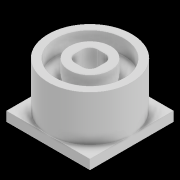
# Autodesk Inventor part: Boton Base
Saved by Autodesk Inventor 2020 (Build 240168000, 168)
## iProperties
Created: 2022-02-20
Part Number: Boton Base
Material: Genérico
Document SubType Name: Modeling
Designer: Alférez
Density: 1 g/cm^3
Appearance: Valor por defecto
Author: Alférez
Autodesk Inventor part; units mm, degrees
ref_plane "YZ Plane" through (0, 0, 0) normal (1, 0, 0) x (0, 1, 0)
ref_plane "XZ Plane" through (0, 0, 0) normal (0, 1, 0) x (-1, 0, 0)
ref_plane "XY Plane" through (0, 0, 0) normal (0, 0, 1) x (1, 0, 0)
sketch "Boceto1" plane through (0, 0, 0) normal (0, 1, 0) x (-1, 0, 0)
  line L0 (0, 0) -> (11, 0)
  line L1 (11, 0) -> (11, -11)
  line L2 (11, -11) -> (0, -11)
  line L3 (0, -11) -> (0, 0)
  dimension "d0" = 11
  dimension "d1" = 11
  constraints: 8 end point, 2 parallel, 1 horizontal, 1 perpendicular
  measures "d0" distance of L1.end L2.end
  measures "d1" distance of L0.end L1.end
extrude "Extrusión1" add sketch "Boceto1" along normal blind 1.25
sketch "Boceto2" plane through (0, 1.25, 0) normal (0, 1, 0) x (1, 0, 0)
  line L0 (-11, 0) -> (0, 0) projected
  line L1 (-11, 11) -> (-11, 0) projected
  line L2 (0, 0) -> (-11, 11)
  line L3 (0, 0) -> (0, 11) projected
  line L4 (0, 11) -> (-11, 0)
  circle A0 centre (-5.5, 5.5) radius 5.5
  dimension "d4" = 11
  constraints: 4 end point, 1 centre point, 1 midpoint
  measures "d4" diameter of A0
extrude "Extrusión2" add sketch "Boceto2" along normal blind 6 contours A0 L4 L2 | A0 L2 L4 | L2 L4 A0 | A0 L4 L2
sketch "Boceto4" plane through (-5.5, 7.25, -5.5) normal (0, 1, 0) x (1, 0, 0)
  line L0 (0, 0) -> (-3, 0)
  line L1 (-3, 0) -> (-3, 1.5)
  line L2 (-3, 1.5) -> (-3, -1.5)
  line L3 (-3, -1.5) -> (-1.5, -1.5)
  line L4 (-1.5, -1.5) -> (-1.5, -3)
  line L5 (-1.5, -3) -> (1.5, -3)
  line L6 (1.5, -3) -> (1.5, -1.5)
  line L7 (1.5, -1.5) -> (3, -1.5)
  line L8 (3, -1.5) -> (3, 1.5)
  line L9 (3, 1.5) -> (1.5, 1.5)
  line L10 (1.5, 1.5) -> (1.5, 3)
  line L11 (1.5, 3) -> (-1.5, 3)
  line L12 (-1.5, 3) -> (-1.5, 1.5)
  line L13 (-3, 1.5) -> (-1.5, 1.5)
  line L14 (-1.5, 1.5) -> (-1.5, -1.5)
  line L15 (1.5, -1.5) -> (1.5, 1.5)
  line L16 (-1.5, 1.5) -> (1.5, 1.5)
  line L17 (1.5, -1.5) -> (-1.5, -1.5)
  point P0 (5.5, -5.5)
  dimension "d7" = 3
  dimension "d8" = 1.5
  dimension "d9" = 3
  dimension "d10" = 1.5
  dimension "d11" = 1.5
  dimension "d12" = 3
  dimension "d13" = 1.5
  dimension "d14" = 1.5
  dimension "d15" = 3
  dimension "d16" = 1.5
  dimension "d17" = 1.5
  dimension "d18" = 3
  constraints: 36 end point, 8 point on line, 6 perpendicular, 1 horizontal, 1 vertical
  measures "d7" distance of L0.start L0.end
  measures "d8" distance of L0.end L1.end
  measures "d9" distance of L1.end L2.end
  measures "d10" distance of L2.end L3.end
  measures "d11" distance of L3.end L4.end
  measures "d12" distance of L4.end L5.end
  measures "d13" distance of L5.end L6.end
  measures "d14" distance of L6.end L7.end
  measures "d15" distance of L7.end L8.end
  measures "d16" distance of L8.end L9.end
  measures "d17" distance of L9.end L10.end
  measures "d18" distance of L10.end L11.end
extrude "Extrusión3" cut sketch "Boceto4" against normal blind 5 contours L14 L16 L15 L17
sketch "Boceto8" plane through (-5.5, 7.25, -5.5) normal (0, 1, 0) x (1, 0, 0)
  circle A0 centre (0, 0) radius 2.75
  circle A1 centre (0, 0) radius 4.5
  point P0 (5.5, -5.5)
  dimension "d47" = 5.5
  dimension "d48" = 9
  constraints: 2 centre point, 1 coincident
  measures "d47" diameter of A0
  measures "d48" diameter of A1
extrude "Extrusión6" cut sketch "Boceto8" against normal blind 2
fillet "Empalme4" radius 1 4 edges at (-7, 4.75, -7) (-4, 4.75, -7) (-4, 4.75, -4) (-7, 4.75, -4)
